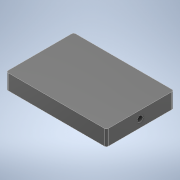
# Autodesk Inventor part: Case - Tampa
Saved by Autodesk Inventor 2021 (Build 250183000, 183)
## iProperties
Created: 2023-01-24
Part Number: Case - Tampa
Material: Plástico PC/ABS
Document SubType Name: Modeling
Designer: nicho
Density: 0.357273 g/cm^3
Appearance: Liso - Preto
Author: nicho
Autodesk Inventor part; units mm, degrees
ref_plane "YZ Plane" through (0, 0, 0) normal (1, 0, 0) x (0, 1, 0)
ref_plane "XZ Plane" through (0, 0, 0) normal (0, 1, 0) x (-1, 0, 0)
ref_plane "XY Plane" through (0, 0, 0) normal (0, 0, 1) x (1, 0, 0)
sketch "Esboço1" plane through (0, 0, 0) normal (0, 1, 0) x (-1, 0, 0)
  line L0 (-26, -17.5) -> (26, -17.5)
  line L1 (26, -17.5) -> (26, 17.5)
  line L2 (26, 17.5) -> (-26, 17.5)
  line L3 (-26, 17.5) -> (-26, -17.5)
  line L4 (-26, -17.5) -> (26, 17.5) construction
  line L5 (26, -17.5) -> (-26, 17.5) construction
  point P0 (0, 0)
  dimension "d0" = 52
  dimension "d1" = 35
  constraints: 12 end point, 2 midpoint, 2 parallel, 1 horizontal, 1 perpendicular
  measures "d0" distance of L2.end L1.end
  measures "d1" distance of L1.end L0.end
extrude "Extrusão1" add sketch "Esboço1" along normal blind 8
fillet "Arredondamento1" radius 1 4 edges at (26, 4, -17.5) (-26, 4, -17.5) (26, 4, 17.5) (-26, 4, 17.5)
sketch "Esboço2" plane through (-26, 0, -16.5) normal (-1, 0, 0) x (0, 0, 1)
  line L0 (0, 8) -> (33, 8) projected
  line L1 (0, 0) -> (33, 0) projected
  point P0 (16.5, 0)
  point P1 (16.5, 4)
  point P2 (16.5, 0)
  dimension "d5" = 4
  constraints: 1 midpoint, 1 vertical alignment
  measures "d5" distance from line of L0 point (16.5, 4)
hole "Furo1" at (-26, 4, 0) direction (1, 0, 0) diameter 3 depth 5 tip angle 118
sketch "Esboço3" plane through (26, 0, 16.5) normal (1, 0, 0) x (0, 0, -1)
  line L0 (0, 8) -> (33, 8) projected
  line L1 (0, 0) -> (33, 0) projected
  point P0 (16.5, 0)
  point P1 (16.5, 4)
  point P2 (16.5, 0)
  dimension "d13" = 4
  constraints: 1 midpoint, 1 vertical alignment
  measures "d13" distance from line of L0 point (16.5, 4)
hole "Furo2" at (26, 4, 0) direction (-1, 0, 0) diameter 3 depth 5 tip angle 118
